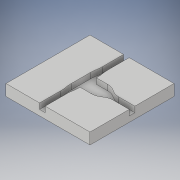
# Autodesk Inventor part: board
Saved by Autodesk Inventor 2019 (Build 230136000, 136)
## iProperties
Created: 2021-08-31
Part Number: board
Material: Generic
Document SubType Name: Modeling
Designer: zachm
Density: 1 g/cm^3
Appearance: Default
Author: zachm
Autodesk Inventor part; units mm, degrees
ref_plane "YZ Plane" through (0, 0, 0) normal (1, 0, 0) x (0, 1, 0)
ref_plane "XZ Plane" through (0, 0, 0) normal (0, 1, 0) x (-1, 0, 0)
ref_plane "XY Plane" through (0, 0, 0) normal (0, 0, 1) x (1, 0, 0)
sketch "Sketch1" plane through (0, 0, 0) normal (0, 1, 0) x (-1, 0, 0)
  line L0 (0, 0) -> (-150, 0)
  line L1 (-150, 0) -> (-150, -150)
  line L2 (-150, -150) -> (0, -150)
  line L3 (0, -150) -> (0, 0)
  line L4 (-58.25, -58) -> (-58.25, -92)
  line L5 (-58.25, -92) -> (-71.75, -92)
  line L6 (-71.75, -92) -> (-71.75, -89.5)
  line L7 (-71.75, -89.5) -> (-91.75, -89.5)
  line L8 (-91.75, -89.5) -> (-91.75, -60.5)
  line L9 (-91.75, -60.5) -> (-71.75, -60.5)
  line L10 (-71.75, -60.5) -> (-71.75, -58)
  line L11 (-71.75, -58) -> (-58.25, -58)
  line L12 (-150, -70) -> (-91.75, -70)
  line L13 (-91.75, -70) -> (-91.75, -80)
  line L14 (-91.75, -80) -> (-150, -80)
  line L15 (-150, -80) -> (-150, -70)
  line L16 (-70, -150) -> (-60, -150)
  line L17 (-60, -150) -> (-60, -92)
  line L18 (-60, -92) -> (-70, -92)
  line L19 (-70, -92) -> (-70, -150)
  line L20 (-60, -58) -> (-70, -58)
  line L21 (-70, -58) -> (-70, 0)
  line L22 (-70, 0) -> (-60, 0)
  line L23 (-60, 0) -> (-60, -58)
  line L24 (-91.75, -70) -> (-121.75, -70)
  line L25 (-91.75, -60.5) -> (-106.75, -60.5) construction
  line L26 (-106.75, -60.5) -> (-106.75, -70) construction
  line L27 (-91.75, -60.5) -> (-106.75, -60.5) construction
  line L28 (-106.75, -60.5) -> (-106.75, -70) construction
  line L29 (-106.75, -70) -> (-121.75, -70) construction
  spline S0 degree 3 poles (-91.75, -60.5) (-106.75, -60.5) (-106.75, -70) (-121.75, -70) knots 1 1 1 1 2 2 2 2
  line L30 (-121.75, -80) -> (-106.75, -80) construction
  line L31 (-106.75, -80) -> (-106.75, -89.5) construction
  line L32 (-106.75, -89.5) -> (-91.75, -89.5) construction
  spline S1 degree 3 poles (-121.75, -80) (-106.75, -80) (-106.75, -89.5) (-91.75, -89.5) knots 1 1 1 1 2 2 2 2
  line L33 (-60, -48) -> (-70, -48) construction
  line L34 (-60, -38) -> (-70, -38) construction
  line L35 (-58.25, -58) -> (-58.25, -48) construction
  line L36 (-58.25, -48) -> (-60, -48) construction
  line L37 (-60, -48) -> (-60, -38) construction
  spline S2 degree 3 poles (-58.25, -58) (-58.25, -48) (-60, -48) (-60, -38) knots 1 1 1 1 2 2 2 2
  line L38 (-70, -38) -> (-70, -48) construction
  line L39 (-70, -48) -> (-71.75, -48) construction
  line L40 (-71.75, -48) -> (-71.75, -58) construction
  spline S3 degree 3 poles (-70, -38) (-70, -48) (-71.75, -48) (-71.75, -58) knots 1 1 1 1 2 2 2 2
  line L41 (-60, -102) -> (-70, -102)
  line L42 (-60, -112) -> (-70, -112)
  line L43 (-58.25, -92) -> (-58.25, -102) construction
  line L44 (-58.25, -102) -> (-60, -102) construction
  line L45 (-60, -102) -> (-60, -112) construction
  spline S4 degree 3 poles (-58.25, -92) (-58.25, -102) (-60, -102) (-60, -112) knots 1 1 1 1 2 2 2 2
  line L46 (-71.75, -92) -> (-71.75, -102) construction
  line L47 (-71.75, -102) -> (-70, -102) construction
  line L48 (-70, -102) -> (-70, -112) construction
  spline S5 degree 3 poles (-71.75, -92) (-71.75, -102) (-70, -102) (-70, -112) knots 1 1 1 1 2 2 2 2
  dimension "d0" = 150
  dimension "d1" = 150
  dimension "d18" = 34
  dimension "d19" = 13.5
  dimension "d20" = 2.5
  dimension "d21" = 20
  dimension "d22" = 29
  dimension "d23" = 20
  dimension "d24" = 2.5
  dimension "d25" = 58.25
  dimension "d26" = 58
  dimension "d27" = 10
  dimension "d28" = 70
  dimension "d29" = 58.25
  dimension "d30" = 10
  dimension "d31" = 1.75
  dimension "d32" = 0
  dimension "d33" = 10
  dimension "d34" = 1.75
  dimension "d35" = 30
  dimension "d36" = 15
  dimension "d37" = 106.75
  dimension "d38" = 121.75
  dimension "d39" = 10
  dimension "d40" = 44
  dimension "d41" = 10
  dimension "d42" = 10
  constraints: 62 end point, 17 point on line, 15 perpendicular, 9 parallel, 8 horizontal, 7 collinear, 6 coincident, 4 vertical, 1 midpoint, 18 other
  measures "d0" distance of L2.end L1.end
  measures "d1" distance of L1.end L0.end
  measures "d18" distance of L4.start L4.end
  measures "d19" distance of L4.end L5.end
  measures "d20" distance of L5.end L6.end
  measures "d21" distance of L6.end L7.end
  measures "d22" distance of L7.end L8.end
  measures "d23" distance of L8.end L9.end
  measures "d24" distance of L9.end L10.end
  measures "d25" distance between parallel lines of L3 L4
  measures "d26" distance between parallel lines of L2 L5
  measures "d27" distance of L12.end L13.end
  measures "d28" distance between parallel lines of L0 L12
  measures "d29" distance of L12.start L12.end
  measures "d30" distance between parallel lines of L19 L17
  measures "d31" distance between parallel lines of L4 L17
  measures "d32" distance between parallel lines of L5 L18
  measures "d33" distance of L21.end L22.end
  measures "d34" distance between parallel lines of L4 L23
  measures "d35" distance of L12.end L24.end
  measures "d36" distance of L8.end L25.end
  measures "d37" distance between parallel lines of L31 L3
  measures "d38" distance from line of L30.start L3
  measures "d39" distance between parallel lines of L34 L33
  measures "d40" distance between parallel lines of L5 L33
  measures "d41" distance between parallel lines of L41 L5
  measures "d42" distance between parallel lines of L42 L41
extrude "Extrusion1" add sketch "Sketch1" along normal blind 10 contours L3 L2 L17 S4 L4 S2 L23 L0 | L21 S3 L10 L9 S0 L12 L1 L0 | L2 L1 L14 S1 L7 L6 S5 L19
sketch "Sketch2" plane through (0, 0, 0) normal (0, -1, 0) x (1, 0, 0)
  line L0 (0, -150) -> (0, 0) projected
  line L1 (150, -80) -> (150, -150) projected
  line L2 (0, 0) -> (150, 0)
  line L3 (150, 0) -> (150, -150)
  line L4 (150, -150) -> (0, -150)
  line L5 (0, -150) -> (0, 0)
  constraints: 8 end point, 2 parallel, 1 horizontal, 1 perpendicular
extrude "Extrusion2" add sketch "Sketch2" along normal blind 10
body "Solid1"
